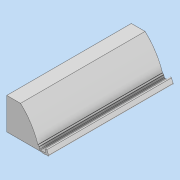
# Autodesk Inventor part: 0 零件
Saved by Autodesk Inventor 2020 (Build 240168000, 168)
## iProperties
Created: 2020-11-03
Part Number: 0 零件
Material: 一般
Document SubType Name: Modeling
Designer: p2013
Density: 1 g/cm^3
Appearance: 預設
Author: p2013
Autodesk Inventor part; units mm, degrees
ref_plane "YZ Plane" through (0, 0, 0) normal (1, 0, 0) x (0, 1, 0)
ref_plane "XZ Plane" through (0, 0, 0) normal (0, 1, 0) x (-1, 0, 0)
ref_plane "XY Plane" through (0, 0, 0) normal (0, 0, 1) x (1, 0, 0)
sketch "草圖3" plane through (0, 0, 0) normal (0, 1, 0) x (-1, 0, 0)
  line L0 (0, 0) -> (0, -300)
  dimension "d15" = 300
  constraints: 2 end point, 1 vertical
  measures "d15" distance of L0.start L0.end
sketch "草圖1" plane through (0, 0, 0) normal (0, 0, 1) x (1, 0, 0)
  line L0 (0, 0) -> (-9.6483, 0) construction
  line L1 (0, 0) -> (0, 8.3837) construction
  line L2 (-7.5155, 4.4979) -> (-7.5, 11.3039)
  arc A0 (-4.2366, 11.9677) -> (-7.5, 11.3039) centre (-5.8, 11.3) ccw
  line L3 (-4.2366, 11.9677) -> (-0.1366, 2.3677)
  arc A1 (-3.1931, 0.8871) -> (-0.1366, 2.3677) centre (-1.7, 1.7) ccw
  line L4 (-3.1931, 0.8871) -> (-4.6931, 0.8871)
  line L5 (-4.6931, 0.8871) -> (-6.6931, 0)
  line L6 (-6.6931, 0) -> (-14.662, 0)
  line L7 (-14.662, 0) -> (-17.0339, 0.8871)
  line L8 (-17.0339, 0.8871) -> (-100.9388, 0.8871)
  line L9 (-21.5255, 4.375) -> (-22.7246, 8.8503)
  line L10 (-23.0602, 9.3678) -> (-25.6826, 11.4969)
  arc A2 (-22.7246, 8.8503) -> (-23.0602, 9.3678) centre (-23.6905, 8.5915) ccw
  line L11 (-13.2, 16.4786) -> (-10.2, 16.4786) construction
  line L12 (-10.2, 16.4786) -> (-10.2, 4.7787) construction
  line L13 (-10.2, 4.7787) -> (-13.2, 4.7787) construction
  line L14 (-13.2, 4.7787) -> (-13.2, 16.4786) construction
  arc A3 (-26.0044, 11.9677) -> (-67.8464, 77.048) centre (-168.8298, -33.868) ccw
  arc A4 (-26.0044, 11.9677) -> (-25.6826, 11.4969) centre (-25.0523, 12.2733) ccw
  line L15 (-67.8464, 77.048) -> (-100.9388, 77.048)
  line L16 (-100.9388, 77.048) -> (-100.9388, 0.8871)
  line L17 (-9.2215, 13) -> (-2.2458, 13) construction
  line L18 (-7.985, 4) -> (-19.985, 3.266)
  arc A5 (-7.985, 4) -> (-7.5155, 4.4979) centre (-8.0155, 4.4991) ccw
  arc A6 (-21.5255, 4.375) -> (-19.985, 3.266) centre (-20.0766, 4.7633) ccw
  point P0 (-25.9139, 11.6848)
  point P1 (-11.7, 4.7787)
  point P2 (-21.314, 3.5858)
  dimension "d0" = 13
  dimension "d4" = 1.7
  dimension "d5" = 1.7
  dimension "d9" = 1
  dimension "d13" = 3
  dimension "d14" = 10
  dimension "d24" = 150
  dimension "d25" = 1
  dimension "d27" = 7.9689
  dimension "d28" = 2
  dimension "d29" = 1.5
  dimension "d31" = 7.5
  dimension "d34" = 75
  dimension "d35" = 23.257
  dimension "d37" = 3.5
  dimension "d38" = 0.5
  dimension "d39" = 12
  dimension "d40" = 9
  dimension "d41" = 1.5
  constraints: 39 end point, 15 point on circle, 14 tangent, 7 centre point, 5 horizontal, 5 point on line, 3 parallel, 2 perpendicular, 1 midpoint, 1 vertical
  measures "d4" radius of A0
  measures "d5" radius of A1
  measures "d9" radius of A2
  measures "d13" distance of L11.start L11.end
  measures "d14" horizontal distance of A1.centre point (-11.7, 4.779)
  measures "d24" radius of A3
  measures "d25" radius of A4
  measures "d27" distance of L5.end L6.end
  measures "d28" horizontal distance of L4.end L5.end
  measures "d29" distance of L4.start L4.end
  measures "d31" distance from line of L2.end L1
  measures "d34" angle of L8 L9
  measures "d35" angle of L3 L2
  measures "d37" angle of L6 L18
  measures "d38" radius of A5
  measures "d39" horizontal distance of L18.start L18.end
  measures "d40" distance from line of L17 L18.start
  measures "d41" radius of A6
sweep "掃掠1" add profiles "草圖1" path "草圖3"
fillet "圓角1" radius 2 3 edges at (-4.6931, 0.8871, -150) (-3.1931, 0.8871, -150) (-6.6931, 0, -150)
